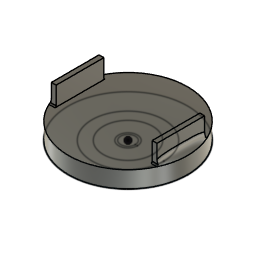
Neck piece bigger attachment v3 (Autodesk Fusion 360 design; units mm, degrees)
Autodesk Fusion 360 part; units mm, degrees
note: some values were not read from the file. Set by a fixed rule: which face or edge a step refers to.
sketch "Sketch1" plane through (0, 0, 0) normal (0, 0, 1) x (1, 0, 0)
  circle A0 centre (0, 0) radius 15.05
  circle A1 centre (0, 0) radius 10.3
  circle A2 centre (0, 0) radius 3.05
  circle A3 centre (0, 0) radius 3.9
  circle A4 centre (0, 0) radius 25
  dimension "d1" = 30.1
  dimension "d2" = 20.6
  dimension "d7" = 6.1
  dimension "d8" = 7.8
  dimension "d9" = 50
  constraint coincident A0.centre A1.centre
  constraint concentric A0 A1
  constraint concentric A0 A2
  constraint concentric A0 A3
  measures "d1" diameter of A0
  measures "d2" diameter of A1
  measures "d7" diameter of A2
  measures "d8" diameter of A3
  measures "d9" diameter of A4
extrude "Extrude1" add sketch "Sketch1" against normal blind 6 contours A0
extrude "Extrude2" add sketch "Sketch1" against normal blind 2 contours A1 | A2 | A3
extrude "Extrude3" add sketch "Sketch1" against normal blind 8 contours A3
extrude "Extrude4" cut 1 faces at (3.5908, -0.3453, -8) along direction (0, 0, 1) blind 7
extrude "Extrude5" add sketch "Sketch1" along normal blind 7 contours A0 | A1 | A2 | A3 | A4
chamfer "Chamfer1" distance 2 angle 45 1 edges at (-9.603, -3.7246, -6)
sketch "Sketch2" plane through (0, 0, 7) normal (0, 0, 1) x (-1, 0, 0)
  circle A0 centre (0, 0) radius 25
  line L0 (20.15, 10) -> (-20.15, 10)
  line L1 (-20.15, 10) -> (-20.15, -10)
  line L2 (-20.15, -10) -> (20.15, -10)
  line L3 (20.15, -10) -> (20.15, 10)
  line L4 (20.15, 10) -> (-20.15, -10) construction
  line L5 (-20.15, 10) -> (20.15, -10) construction
  line L6 (-20.15, 10) -> (-22.15, 10)
  line L7 (-22.15, 10) -> (-22.15, -10)
  line L8 (-22.15, -10) -> (-20.15, -10)
  line L9 (-20.15, -10) -> (-20.15, 10)
  line L10 (20.15, 10) -> (22.15, 10)
  line L11 (22.15, 10) -> (22.15, -10)
  line L12 (22.15, -10) -> (20.15, -10)
  line L13 (20.15, -10) -> (20.15, 10)
  dimension "d17" = 40.3
  dimension "d18" = 20
  dimension "d19" = 2
  dimension "d20" = 20
  dimension "d21" = 2
  dimension "d22" = 20
  constraint horizontal L0
  constraint perpendicular L0 L1
  constraint parallel L0 L2
  constraint parallel L1 L3
  constraint coincident L4 A0.centre
  constraint coincident L5 A0.centre
  constraint coincident A0.centre origin
  constraint horizontal L6
  constraint vertical L7
  constraint horizontal L8
  constraint vertical L9
  constraint horizontal L10
  constraint vertical L11
  constraint horizontal L12
  constraint vertical L13
  measures "d17" distance of L1.end L2.end
  measures "d18" distance of L0.end L1.end
  measures "d19" distance of L0.end L6.end
  measures "d20" distance of L0.end L1.end
  measures "d21" distance of L0.start L10.end
  measures "d22" distance of L0.start L2.end
extrude "Extrude6" add sketch "Sketch2" along normal blind 8 contours L3 L10 L11 L12 L13 | L1 L6 L7 L8 L9
fillet "Fillet1" radius 3 2 edges at (-22.15, 0, 7) (22.15, 0, 7)
fillet "Fillet2" radius 0.5 4 edges at (-21.5314, 10, 7) (21.5314, 10, 7) (-21.5314, -10, 7) (21.5314, -10, 7)
extrude "Extrude7" cut 2 faces at (8.1283, -0.5117, -2) (-0.679, -0.4952, -2) along direction (0, 0, 1) blind 1
extrude "Extrude8" cut 3 faces at (8.1283, -0.5117, -1) (3.5908, -0.3453, -1) (-0.679, -0.4952, -1) along direction (0, 0, 1) blind 0.5
named bodies: "Neck Connetion"
